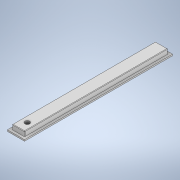
# Autodesk Inventor part: enclosureTop
Saved by Autodesk Inventor 2020 (Build 240168000, 168)
## iProperties
Created: 2020-04-01
Part Number: enclosureTop
Material: Generic
Document SubType Name: Modeling
Designer: Clevo
Density: 1 g/cm^3
Appearance: Default
Author: Clevo
Autodesk Inventor part; units mm, degrees
ref_plane "YZ Plane" through (0, 0, 0) normal (1, 0, 0) x (0, 1, 0)
ref_plane "XZ Plane" through (0, 0, 0) normal (0, 1, 0) x (-1, 0, 0)
ref_plane "XY Plane" through (0, 0, 0) normal (0, 0, 1) x (1, 0, 0)
sketch "Sketch1" plane through (0, 0, 0) normal (0, 1, 0) x (-1, 0, 0)
  line L0 (-12.7, -148.5) -> (12.7, -148.5)
  line L1 (12.7, -148.5) -> (12.7, 148.5)
  line L2 (12.7, 148.5) -> (-12.7, 148.5)
  line L3 (-12.7, 148.5) -> (-12.7, -148.5)
  line L4 (-12.7, -148.5) -> (12.7, 148.5) construction
  line L5 (12.7, -148.5) -> (-12.7, 148.5) construction
  point P0 (0, 0)
  dimension "d0" = 25.4
  dimension "d1" = 297
  constraints: 12 end point, 2 midpoint, 2 parallel, 1 horizontal, 1 perpendicular
  measures "d0" distance of L1.end L2.end
  measures "d1" distance of L0.end L1.end
extrude "Extrusion1" add sketch "Sketch1" along normal blind 10
sketch "Sketch2" plane through (0, 0, 0) normal (0, -1, 0) x (1, 0, 0)
  line L0 (12.7, -148.5) -> (-12.7, -148.5) projected
  line L1 (12.7, 148.5) -> (12.7, -148.5) projected
  line L2 (-12.7, 148.5) -> (12.7, 148.5) projected
  line L3 (-12.7, -148.5) -> (-12.7, 148.5) projected
  line L4 (17.7, -153.5) -> (-17.7, -153.5)
  line L5 (-17.7, -153.5) -> (-17.7, 153.5)
  line L6 (-17.7, 153.5) -> (17.7, 153.5)
  line L7 (17.7, 153.5) -> (17.7, -153.5)
  point P0 (0, 0)
  dimension "d4" = 5
  constraints: 8 end point, 3 other
  measures "d4" distance between parallel lines of L1 L7
extrude "Extrusion2" add sketch "Sketch2" along normal blind 3 contours L0 L3 L2 L1 | L4 L5 L6 L7
sketch "Sketch3" plane through (0, 10, 0) normal (0, 1, 0) x (1, 0, 0)
  line L0 (12.7, 148.5) -> (-12.7, 148.5) projected
  line L1 (-12.7, 148.5) -> (-12.7, -148.5) projected
  line L2 (-12.7, -148.5) -> (12.7, -148.5) projected
  line L3 (12.7, -148.5) -> (12.7, 148.5) projected
  circle A0 centre (0, -130) radius 5
  point P0 (0, 0)
  dimension "d7" = 10
  dimension "d8" = 130
  constraints: 1 centre point, 1 vertical alignment
  measures "d7" diameter of A0
  measures "d8" distance of point (0, 0) A0.centre
extrude "Extrusion3" cut sketch "Sketch3" against normal through all contours A0
fillet "Fillet1" radius 1 8 edges at (12.7, 5, 148.5) (-12.7, 5, 148.5) (12.7, 5, -148.5) (-12.7, 5, -148.5) (0, 10, -148.5) (-12.7, 10, 0) (12.7, 10, 0) (0, 10, 148.5)
body "Solid1"
